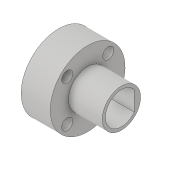
# Autodesk Inventor part: Our omiwheelinsert
Saved by Autodesk Inventor 2020 (Build 240168000, 168)
## iProperties
Created: 2019-09-23
Part Number: Our omiwheelinsert
Material: Generic
Document SubType Name: Modeling
Designer: ball
Density: 1 g/cm^3
Appearance: Default
Author: ball
Autodesk Inventor part; units mm, degrees
ref_plane "YZ Plane" through (0, 0, 0) normal (1, 0, 0) x (0, 1, 0)
ref_plane "XZ Plane" through (0, 0, 0) normal (0, 1, 0) x (-1, 0, 0)
ref_plane "XY Plane" through (0, 0, 0) normal (0, 0, 1) x (1, 0, 0)
sketch "Sketch1" plane through (0, 0, 0) normal (1, 0, 0) x (0, 1, 0)
  circle A0 centre (0, 0) radius 7.7343
  dimension "d0" = 15.4686
  constraints: 1 centre point, 1 coincident
  measures "d0" diameter of A0
extrude "Extrusion1" add sketch "Sketch1" along normal blind 6.0198
sketch "Sketch2" plane through (6.0198, 0, 0) normal (1, 0, 0) x (0, 0, -1)
  circle A0 centre (0, 0) radius 3.9624
  dimension "d3" = 7.9248
  constraints: 1 centre point, 1 coincident
  measures "d3" diameter of A0
extrude "Extrusion2" add sketch "Sketch2" along normal blind 6.985
sketch "Sketch3" plane through (0, 0, 0) normal (-1, 0, 0) x (0, 0, 1)
  arc A0 (-2.6416, -2.0232) -> (-2.6416, 2.0232) centre (0, 0) ccw
  line L0 (-2.6416, -2.0232) -> (-2.6416, 2.0232)
  dimension "d6" = 6.6548
  constraints: 2 end point, 2 point on circle, 1 centre point, 1 coincident, 1 vertical
  measures "d6" diameter of A0
extrude "Extrusion3" cut sketch "Sketch3" against normal through all
sketch "Sketch4" plane through (0, 0, 0) normal (-1, 0, 0) x (0, 0, 1)
  circle A0 centre (-4.2426, 4.2418) radius 1.15
  circle A1 centre (0, 0) radius 6 construction
  circle A2 centre (-4.2418, -4.2426) radius 1.15
  circle A3 centre (4.2426, -4.2418) radius 1.15
  circle A4 centre (4.2418, 4.2426) radius 1.15
  dimension "d12" = 2.3
  dimension "d21" = 12
  dimension "d24" = 360
  constraints: 5 centre point, 1 coincident, 9 other
  measures "d12" diameter of A0
  measures "d21" diameter of A1
extrude "Extrusion4" cut sketch "Sketch4" against normal through all
sketch "Sketch5" plane through (0, -2.0232, -2.6416) normal (0, 0, 1) x (1, 0, 0)
  circle A0 centre (3.0099, 2.0232) radius 1.45
  line L0 (6.0198, -5.7111) -> (6.0198, 9.7575) projected
  line L1 (0, 9.7575) -> (0, -5.7111) projected
  line L2 (6.0198, 5.9856) -> (13.0048, 5.9856) construction
  line L3 (13.0048, -1.9392) -> (13.0048, 5.9856) construction
  line L4 (6.0198, 5.9856) -> (6.0198, -1.9392) construction
  line L5 (0, 9.7575) -> (6.0198, 9.7575) construction
  line L6 (0, -5.7111) -> (6.0198, -5.7111) construction
  point P0 (0, 2.0232)
  dimension "d26" = 2.9
  dimension "d27" = 6.0198
  dimension "d28" = 3.0099
  dimension "d29" = 15.4686
  dimension "d30" = 7.7343
  constraints: 1 centre point
  measures "d26" diameter of A0
  measures "d27" distance between parallel lines of L0 L1
  measures "d28" distance from line of L1 A0.centre
  measures "d29" distance between parallel lines of L6 L5
  measures "d30" distance from line of L5 A0.centre
extrude "Extrusion5" cut sketch "Sketch5" against normal through all
equation "\"d28\" = 0.5 * d27"
equation "\"d30\" = 0.5 * d29"
body "Solid1"
